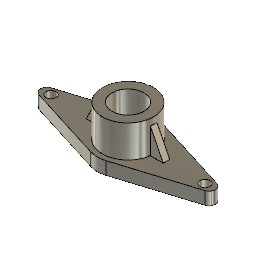
Semana3_Desafio3 v1 (Autodesk Fusion 360 design; units mm, degrees)
Autodesk Fusion 360 part; units mm, degrees
sketch "Sketch1" plane through (0, 0, 0) normal (0, 0, 1) x (1, 0, 0)
  line L0 (0, -25) -> (-80, 0)
  line L1 (-80, 0) -> (0, 25)
  line L2 (80, 0) -> (0, 25)
  line L3 (80, 0) -> (0, -25)
extrude "Extrude1" add sketch "Sketch1" along normal blind 10 makes body 1
fillet "Fillet3" radius 20 1 edges at (0, 25, 5) on bodies 1
fillet "Fillet4" radius 20 1 edges at (0, -25, 5) on bodies 1
sketch "Sketch5" plane through (0, 0, 10) normal (0, 0, 1) x (-1, 0, 0)
  arc A0 (5.9655, 23.1358) -> (-5.9655, 23.1358) centre (0, 4.0462) ccw
  line L0 (-5.9655, 23.1358) -> (-80, 0)
  line L1 (-80, 0) -> (-5.9655, -23.1358)
  arc A1 (-5.9655, -23.1358) -> (5.9655, -23.1358) centre (0, -4.0462) ccw
  line L2 (5.9655, -23.1358) -> (80, 0)
  line L3 (80, 0) -> (5.9655, 23.1358)
  circle A2 centre (0, 0) radius 20
  circle A3 centre (0, 0) radius 12.5
  dimension "d19" = 25
  constraint coincident A2.centre A3.centre
  measures "d19" diameter of A3
extrude "Extrude5" add sketch "Sketch5" along normal blind 25 contours A2 bodies 1
extrude "Extrude6" cut 1 faces at (-0.8448, -2.1525, 10) along direction (0, 0, -1) blind 60 on bodies 1 bodies 1
sketch "Sketch8" plane through (0, 0, 0) normal (0, 1, 0) x (1, 0, 0)
  line L0 (-20, -30) -> (-30, -10)
  line L1 (-30, -10) -> (-20, -10)
  line L2 (-20, -10) -> (-20, -30)
  line L3 (20, -30) -> (30, -10)
  line L4 (30, -10) -> (20, -10)
  line L5 (20, -10) -> (20, -30)
  constraint horizontal L1
  constraint perpendicular L1 L2
  constraint perpendicular L2 L4
  constraint perpendicular L4 L5
extrude "Extrude8" add sketch "Sketch8" along normal blind 2.5 separate body makes body 2 at (-23.3333, 0, 16.6667) makes body 3 at (23.3333, 0, 16.6667)
extrude "Extrude9" add 1 faces at (-23.3333, 0, 16.6667) along direction (0, -1, 0) blind 2.5 on bodies 2 bodies 2 3 1
extrude "Extrude10" add 1 faces at (23.3333, 0, 16.6667) along direction (0, -1, 0) blind 2.5 on bodies 3 bodies 3 2
fillet "Fillet5" radius 5 1 edges at (-80, 0, 5) on bodies 3
fillet "Fillet6" radius 5 1 edges at (80, 0, 5) on bodies 3
sketch "Sketch9" plane through (0, 0, 10) normal (0, 0, 1) x (-1, 0, 0)
  arc A0 (-20, 0) -> (20, 0) centre (0, 0) ccw
  line L0 (-20, 0) -> (-20, -2.5)
  line L1 (-20, -2.5) -> (-30, -2.5)
  line L2 (-30, -2.5) -> (-30, 2.5)
  line L3 (-30, 2.5) -> (-20, 2.5)
  line L4 (-20, 2.5) -> (-20, 0)
  arc A1 (20, 0) -> (-20, 0) centre (0, 0) ccw
  line L5 (20, 0) -> (20, 2.5)
  line L6 (20, 2.5) -> (30, 2.5)
  line L7 (30, 2.5) -> (30, -2.5)
  line L8 (30, -2.5) -> (20, -2.5)
  line L9 (20, -2.5) -> (20, 0)
  arc A2 (-64.7283, 4.7724) -> (-64.7283, -4.7724) centre (-63.2369, 0) ccw
  line L10 (-64.7283, -4.7724) -> (-5.9655, -23.1358)
  arc A3 (-5.9655, -23.1358) -> (5.9655, -23.1358) centre (0, -4.0462) ccw
  line L11 (5.9655, -23.1358) -> (64.7283, -4.7724)
  arc A4 (64.7283, -4.7724) -> (64.7283, 4.7724) centre (63.2369, 0) ccw
  line L12 (64.7283, 4.7724) -> (5.9655, 23.1358)
  arc A5 (5.9655, 23.1358) -> (-5.9655, 23.1358) centre (0, 4.0462) ccw
  line L13 (-5.9655, 23.1358) -> (-64.7283, 4.7724)
  circle A6 centre (60, 0) radius 4
  circle A7 centre (-60, 0) radius 4
  dimension "d34" = 8
  dimension "d35" = 8
  measures "d34" diameter of A6
  measures "d35" diameter of A7
extrude "Extrude11" cut sketch "Sketch9" against normal blind 40 contours A6 | A7 bodies 3
